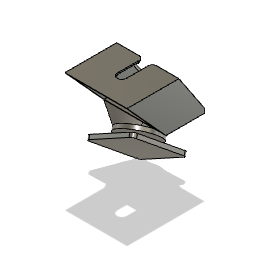
dripdown-orange30 (Autodesk Fusion 360 design; units mm, degrees)
Autodesk Fusion 360 part; units mm, degrees
note: some values were not read from the file. Chosen so that the rebuilt part matches the saved one: which sketch regions a step uses; which pieces of a blend or face edit are solid.
sketch "スケッチ1" plane through (0, 0, 0) normal (0, 1, 0) x (1, 0, 0)
  line L0 (24, -20) -> (-24, -20)
  line L1 (-24, -20) -> (-24, 20)
  line L2 (-24, 20) -> (24, 20)
  line L3 (24, 20) -> (24, -20)
  line L4 (24, -20) -> (-24, 20) construction
  line L5 (-24, -20) -> (24, 20) construction
  line L6 (-21, -20) -> (-21, 20)
  line L7 (21, 20) -> (21, -20)
  line L8 (-3.55, 0) -> (-3.55, 20)
  line L9 (3.55, 0) -> (3.55, 20)
  arc A0 (-3.55, 0) -> (3.55, 0) centre (0, 0) ccw
  line L10 (-24, 20) -> (24, 20)
  line L11 (24, 20) -> (24, 40)
  line L12 (24, 40) -> (-24, 40)
  line L13 (-24, 40) -> (-24, 20)
  dimension "d1" = 48
  dimension "d2" = 40
  dimension "d6" = 3
  dimension "d7" = 3
  dimension "d79" = 20
  constraint perpendicular L0 L1
  constraint parallel L0 L2
  constraint parallel L1 L3
  constraint horizontal L0
  constraint coincident L4 A0.centre
  constraint coincident L5 A0.centre
  constraint coincident A0.centre origin
  constraint coincident L0 L6.start
  constraint coincident L2 L6.end
  constraint perpendicular L2 L6
  constraint coincident L2 L7.start
  constraint coincident L0 L7.end
  constraint perpendicular L0 L7
  constraint coincident L2 L8.end
  constraint perpendicular L2 L8
  constraint coincident L2 L9.end
  constraint perpendicular L2 L9
  constraint horizontal L10
  constraint vertical L11
  constraint horizontal L12
  constraint vertical L13
  constraint collinear L3 L11
  measures "d1" distance of L1.end L2.end L0.start
  measures "d2" distance of L0.end L1.end L0.start
  measures "d6" distance of L1 L6
  measures "d7" distance of L3 L7
  measures "d79" distance of L1.end L12.end
extrude "押し出し1" add sketch "スケッチ1" along normal blind 3 contours L0 L2 L3 L7 L10 | L0 L2 L6 L7 L8 L9 A0 L10 | L0 L1 L2 L6 L10 makes body 1
extrude "押し出し2" add sketch "スケッチ1" against normal blind 30 contours L0 L2 L3 L7 L10 | L0 L1 L2 L6 L10 bodies 1
extrude "押し出し7" add sketch "スケッチ1" along normal blind 3 from surface at -30 bodies 1
sketch "スケッチ7" plane through (-24, 0, 0) normal (-1, 0, 0) x (0, 0, 1)
  line L0 (20, -30) -> (20, 3)
  line L1 (20, 3) -> (-20, 3)
  line L2 (-20, 3) -> (-20, -27)
  line L3 (-40, -30) -> (20, -30)
  line L4 (15, -25) -> (15, -2)
  line L5 (15, -2) -> (-15, -2)
  line L6 (-15, -2) -> (-15, -25)
  line L7 (-15, -25) -> (15, -25)
  line L8 (-20, -27) -> (-40, -27)
  line L9 (-40, -27) -> (-40, -30)
  line L10 (-20, 3) -> (-40, -27)
  line L11 (20, 3) -> (-10, -30)
  constraint parallel L0 L4
  constraint parallel L1 L5
  constraint parallel L2 L6
  constraint parallel L3 L7
  constraint coincident L1.end L2.start
  constraint coincident L8.end L9.start
  constraint coincident L0.end L1.start
  constraint midpoint L3 L11.end
extrude "押し出し8" add sketch "スケッチ7" against normal blind 3 contours L2 L8 L10 bodies 1
extrude "押し出し9" add sketch "スケッチ7" along normal blind 3 from surface at -48 contours L2 L8 L10 bodies 1
ref_plane "作業平面5" through (22.5, -50, 0) normal (0, -1, 0) x (0, 0, -1)
sketch "スケッチ4" plane through (21, -50, 0) normal (0, -1, 0) x (1, 0, 0)
  line L0 (20, 20) -> (-20, 20)
  line L1 (-20, 20) -> (-20, -20)
  line L2 (20, -20) -> (20, 20)
  line L3 (20, 20) -> (-20, -20) construction
  line L4 (-20, 20) -> (20, -20) construction
  line L5 (-3.55, -20) -> (-3.55, 0) construction
  arc A0 (3.55, 0) -> (-3.55, 0) centre (0, 0) ccw construction
  line L6 (3.55, 0) -> (3.55, -20) construction
  line L7 (-20, -20) -> (-3.55, -20)
  line L8 (3.55, -20) -> (20, -20)
  circle A1 centre (0, 0) radius 15
  circle A2 centre (0, 0) radius 3.25
  line L9 (-3.55, -20) -> (3.55, -20)
  dimension "d23" = 40
  dimension "d24" = 40
  dimension "d25" = 7.1
  dimension "d26" = 30
  dimension "d27" = 6.5
  constraint perpendicular L0 L1
  constraint parallel L0 L7
  constraint parallel L1 L2
  constraint horizontal L0
  constraint coincident L3 A0.centre
  constraint coincident L4 A0.centre
  constraint coincident A0.centre A1.centre
  constraint tangent A0 L6
  constraint collinear L7 L8
  constraint concentric A1 A2
  constraint perpendicular L6 L9
  measures "d23" distance of L1.end L2.start
  measures "d24" distance of L0.end L1.end
  measures "d25" distance of L5.start L6.end
  measures "d26" diameter of A1
  measures "d27" diameter of A2
extrude "押し出し4" add sketch "スケッチ4" along normal blind 3 separate body contours A1 | A2 makes body 2
extrude "押し出し5" add sketch "スケッチ4" along normal blind 7 contours A2 bodies 2
extrude "押し出し6" add sketch "スケッチ4" along normal blind 3 from surface at 7 contours L0 L1 L2 L7 L8 L9 | A1 | A2 bodies 2
move_body "移動1" bodies 2 to x (1, 0, 0) y (0, 1, 0) z (0, 0, 1) at (-20.8977, 0, 2.0699)
sketch "スケッチ5" plane through (0, -50, 0) normal (0, 1, 0) x (-1, 0, 0)
  circle A0 centre (-0.1023, 2.0699) radius 15
  line L0 (14.8977, 2.0699) -> (-15.1023, 2.0699) construction
  line L1 (0, -16) -> (0, 21) construction
  constraint coincident A0 L0.start
  constraint coincident A0 L0.end
  constraint horizontal L0
  constraint vertical L1
move_body "移動5" bodies 2 to x (0.819152, 0.573576, 0) y (-0.573576, 0.819152, 0) z (0, 0, 1) at (-28.6788, -9.0424, 0)
move_body "移動6" bodies 2 to x (1, 0, 0) y (0, 0.819152, -0.573576) z (0, 0.573576, 0.819152) at (0, -10.2297, -28.3045)
move_body "移動7" bodies 2 to x (1, 0, 0) y (0, 1, 0) z (0, 0, 1) at (0, -10, 0)
move_body "移動8" bodies 2 to x (1, 0, 0) y (0, 1, 0) z (0, 0, 1) at (-4, -5, -5)
move_body "移動9" bodies 2 to x (1, 0, 0) y (0, 1, 0) z (0, 0, 1) at (0, -2, 0)
move_body "移動10" bodies 2 to x (1, 0, 0) y (0, 1, 0) z (0, 0, 1) at (-40, 0, 0)
move_body "移動11" bodies 2 to x (1, 0, 0) y (0, 1, 0) z (0, 0, 1) at (0, 0, -35)
move_body "移動12" bodies 2 to x (1, 0, 0) y (0, 1, 0) z (0, 0, 1) at (0, -25, 0)
move_body "移動13" bodies 2 to x (1, 0, 0) y (0, 1, 0) z (0, 0, 1) at (5, 0, 0)
move_body "移動14" bodies 2 to x (0.939693, 0, 0.34202) y (0, 1, 0) z (-0.34202, 0, 0.939693) at (-22.806, 0, 14.0643)
move_body "移動15" bodies 2 to x (1, 0, 0) y (0, 1, 0) z (0, 0, 1) at (10, 0, 0)
move_body "移動16" bodies 2 to x (1, 0, 0) y (0, 1, 0) z (0, 0, 1) at (15, 0, 0)
move_body "移動17" bodies 2 to x (1, 0, 0) y (0, 1, 0) z (0, 0, 1) at (0, 30, 0)
sketch "スケッチ12" plane through (0, -30, 0) normal (0, -1, 0) x (1, 0, 0)
  line L0 (24, 20) -> (-24, 20)
  line L1 (-24, 20) -> (-24, -40)
  line L2 (-24, -40) -> (24, -40)
  line L3 (24, -40) -> (24, 20)
  line L4 (-24, -40) -> (6, -40)
  line L5 (6, -40) -> (6, -10)
  line L6 (6, -10) -> (-24, -10)
  line L7 (-24, -10) -> (-24, -40)
  line L8 (-19, -35) -> (1, -35)
  line L9 (1, -35) -> (1, -15)
  line L10 (1, -15) -> (-19, -15)
  line L11 (-19, -15) -> (-19, -35)
  dimension "d85" = 30
  dimension "d86" = 30
  dimension "d87" = -5
  constraint horizontal L4
  constraint vertical L5
  constraint horizontal L6
  constraint vertical L7
  constraint coincident L1.end L2.start
  measures "d85" distance of L1.end L6.end
  measures "d86" distance of L1.end L4.end
sketch "スケッチ13" plane through (4.2408, -7.5223, 7.1487) normal (-0.378289, 0.67101, -0.637686) x (-0.860054, 0, 0.510202)
  circle A0 centre (0.5811, -73.4099) radius 15
  circle A1 centre (0.5811, -73.4099) radius 5
  dimension "d88" = -10
loft "ロフト6" add profiles "スケッチ13", "スケッチ12" section 1 contours A0 | A1 section 2 contours L1 L2 L4 L5 L6 L7 bodies 1 2
extrude "押し出し11" cut sketch "スケッチ7" against normal blind 48 contours L0 L3 L4 L7 L11 | L4 L7 L11 bodies 1
fillet "フィレット4" radius 3 2 edges at (3.55, 1.5, -20) (-3.55, 1.5, -20) on bodies 1
fillet "フィレット5" radius 3 2 edges at (-6.1334, -46.7871, -14.6844) (-41.4243, -65.5809, -13.5251) on bodies 1 2
fillet "フィレット6" radius 2 7 edges at (-13.775, 0, -20) (-4.4287, 0, -19.1213) (-3.55, 0, -8.5) (0, 0, 3.55) (3.55, 0, -8.5) (4.4287, 0, -19.1213) (13.775, 0, -20) on bodies 1
fillet "フィレット7" radius 2 2 edges at (21, -12, -30) (-21, -12, -30) on bodies 1
fillet "フィレット8" radius 2 2 edges at (5.0732, -69.7301, -45.4744) (-30.2176, -88.524, -44.3151) on bodies 1 2
